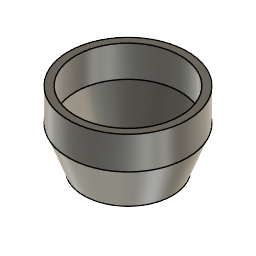
Ghiveci (Autodesk Fusion 360 design; units mm, degrees)
part number: 2026-06-05-21-46-32-778
Autodesk Fusion 360 part; units mm, degrees
sketch "Sketch1" plane through (0, 0, 0) normal (0, 1, 0) x (1, 0, 0)
  line L0 (-50, -70) -> (-50, -40)
  line L1 (-35, 0) -> (-42.3108, 0)
  line L2 (0, 0) -> (0, -7)
  line L3 (-56.8453, -38.7587) -> (-42.3108, 0)
  line L4 (0, 0) -> (-35, 0)
  line L5 (0, -7) -> (-37.625, -7)
  line L6 (-37.625, -7) -> (-50, -40)
  line L7 (-50, -70) -> (-56.8453, -70)
  line L8 (-56.8453, -38.7587) -> (-56.8453, -70)
  dimension "d1" = 35
  dimension "d2" = 56.8453
  dimension "d3" = 70
  dimension "d4" = 6.8453
  dimension "d5" = 7
  dimension "d6" = 110.556
  dimension "d7" = 6.8453
  dimension "d8" = 37.625
  constraint coincident L2.start L4.start
  constraint horizontal L4
  constraint parallel L1 L4
  constraint perpendicular L7 L8
  constraint perpendicular L0 L7
  constraint parallel L4 L7
  constraint perpendicular L2 L4
  constraint perpendicular L2 L5
  constraint parallel L3 L6
  measures "d1" distance of L2.start L1.start
  measures "d2" distance of L2.start L8
  measures "d3" distance of L4 L7
  measures "d4" distance of L0 L8
  measures "d5" distance of L2.end L2.start
  measures "d6" angle of L5 L6
  measures "d7" distance of L3 L6
  measures "d8" distance of L5.end L2
revolve "Revolve1" add sketch "Sketch1" angle 360 about axis through (0, 0, 1.75) along (0, 0, 1)
